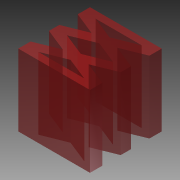
# Autodesk Inventor part: Jack
Saved by Autodesk Inventor 2014 SP1 (Build 180222100, 222)
## iProperties
Created: 2017-01-20
Part Number: Jack
Material: Generic
Document SubType Name: Modeling
Designer: danielsikar
Density: 1 g/cm^3
Appearance: Dark Red
Author: danielsikar
Autodesk Inventor part; units mm, degrees
ref_plane "YZ Plane" through (0, 0, 0) normal (1, 0, 0) x (0, 1, 0)
ref_plane "XZ Plane" through (0, 0, 0) normal (0, 1, 0) x (-1, 0, 0)
ref_plane "XY Plane" through (0, 0, 0) normal (0, 0, 1) x (1, 0, 0)
sketch "Sketch1" plane through (0, 0, 0) normal (0, 0, 1) x (1, 0, 0)
  line L0 (0, 0) -> (30, 0) construction
  line L1 (30, 0) -> (30, 30) construction
  line L2 (30, 30) -> (0, 30) construction
  line L3 (0, 30) -> (0, 0) construction
  line L4 (0, 0) -> (30, 0)
  line L5 (36.8144, 0) -> (36.8144, 3)
  line L6 (0, 3) -> (0, 0)
  line L7 (0, 30) -> (30, 30)
  line L8 (30, 30) -> (30, 27)
  line L9 (24.6148, 27) -> (5.3852, 27)
  line L10 (0, 27) -> (0, 30)
  line L11 (0, 15) -> (30, 15) construction
  line L12 (30, 27) -> (0, 15) construction
  line L13 (12.3074, 22.077) -> (30, 15) construction
  line L14 (30, 27) -> (30, 3)
  line L15 (0, 27) -> (0, 3)
  line L16 (24.6148, 27) -> (15, 23.1541)
  line L17 (9.6148, 21) -> (0, 17.1541)
  line L18 (30, 24.8459) -> (20.3852, 21)
  line L19 (5.3852, 27) -> (15, 23.1541)
  line L20 (20.3852, 21) -> (30, 17.1541)
  line L21 (0, 24.8459) -> (9.6148, 21)
  line L22 (20.3852, 9) -> (30, 5.1541)
  line L23 (0, 12.8459) -> (9.6148, 9)
  line L24 (15, 6.8459) -> (24.6148, 3)
  line L25 (24.6148, 15) -> (15, 11.1541)
  line L26 (9.6148, 9) -> (0, 5.1541)
  line L27 (0, 15) -> (15, 9) construction
  line L28 (17.6926, 7.923) -> (30, 3) construction
  line L29 (15, 18.8459) -> (5.3852, 15)
  line L30 (5.3852, 15) -> (15, 11.1541)
  line L31 (36.8144, 3) -> (35.3852, 3)
  line L32 (24.6148, 3) -> (5.3852, 3)
  line L33 (30, 0) -> (30, 3)
  line L34 (30, 15) -> (27.3074, 13.923) construction
  line L35 (15, 9) -> (0, 3) construction
  line L36 (15, 18.8459) -> (24.6148, 15)
  line L37 (30, 12.8459) -> (20.3852, 9)
  line L38 (17.6926, 7.923) -> (5.3852, 3)
  line L39 (0, 9) -> (0, 37.598)
  line L40 (0, 24.8459) -> (0, 17.1541)
  dimension "d0" = 30
  dimension "d1" = 30
  dimension "d2" = 3
  dimension "d3" = 3
  constraints: 82 end point, 32 parallel, 15 point on line, 4 collinear, 3 horizontal, 3 perpendicular, 2 midpoint
  measures "d0" distance of L2.end L1.end
  measures "d1" distance of L0.end L1.end
  measures "d2" distance of L5.end L5.start
  measures "d3" distance of L7.end L8.end
extrude "Extrusion1" add sketch "Sketch1" along normal blind 30 contours L6 L15 L26 L23 L17 L21 L10 L7 L8 L14 L18 L20 L37 L22 L33 L4
body "Solid1"
